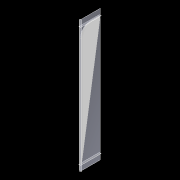
# Autodesk Inventor part: 路徑
Saved by Autodesk Inventor 2020 (Build 240168000, 168)
## iProperties
Created: 2021-04-14
Part Number: 路徑
Material: 一般
Document SubType Name: Modeling
Designer: 88690
Density: 1 g/cm^3
Appearance: 預設
Author: 88690
Autodesk Inventor part; units mm, degrees
sketch "草圖1" plane through (0, 0, 0) normal (1, 0, 0) x (0, 1, 0)
  line L0 (0, 0) -> (674.096, -106.071)
  line L1 (0, 0) -> (614.096, 0)
  line L2 (674.096, -106.071) -> (674.096, -60)
  line L3 (674.096, -106.071) -> (0, -106.071) construction
  line L4 (0, 0) -> (0, -106.071)
  arc A0 (674.096, -60) -> (614.096, 0) centre (614.096, -60) ccw
  dimension "d0" = 106.071
  dimension "d1" = 674.096
  dimension "d2" = 60
  constraints: 10 end point, 2 horizontal, 2 point on circle, 2 tangent, 2 vertical, 1 centre point
  measures "d0" distance of L0.start L3.end
  measures "d1" distance of L0.end L3.end
  measures "d2" radius of A0
extrude "擠出1" add sketch "草圖1" along normal mid plane 10
ref_plane "工作平面1" through (0, 674.096, 0) normal (0, 1, 0) x (-1, 0, 0)
fillet "圓角1" radius 5 6 edges at (-5, 656.5224, -17.5736) (-5, 307.048, 0) (-5, 674.096, -83.0355) (5, 307.048, 0) (5, 674.096, -83.0355) (5, 656.5224, -17.5736)
